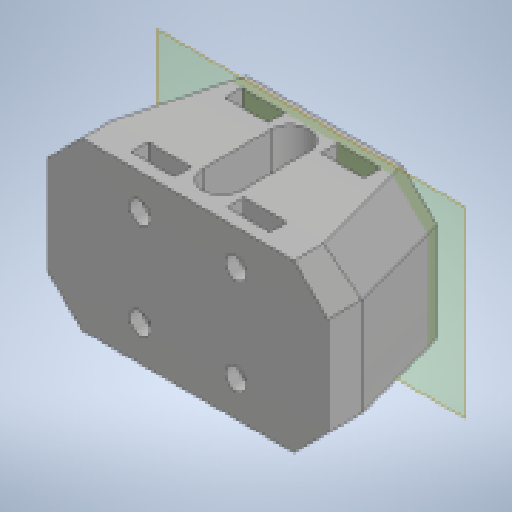
# Autodesk Inventor part: MCP-V
Saved by Autodesk Inventor 2026 (Build 300175050, 175E)
## iProperties
Created: 2025-12-08
Part Number: MCP-V
Material: Genérico
Document SubType Name: Modeling
Designer: user
Density: 1 g/cm^3
Appearance: Gris claro
Author: user
Autodesk Inventor part; units mm, degrees
ref_plane "YZ Plane" through (0, 0, 0) normal (1, 0, 0) x (0, 1, 0)
ref_plane "Plano de trabajo1" through (-13.3, -9.8, -7.75) normal (0, 0, 1) x (1, 0, 0)
ref_plane "Plano de trabajo2" through (-13.3, -9.8, -8.0345) normal (0, 0, 1) x (1, 0, 0)
sketch "Boceto1" plane through (0, 0, 0) normal (0, 0, 1) x (1, 0, 0)
  line L0 (13.3, 9.8) -> (-13.3, 9.8) projected
  line L1 (-13.3, -9.8) -> (-13.3, 9.8) projected
  line L2 (-13.3, -9.8) -> (13.3, -9.8) projected
  line L3 (13.3, 9.8) -> (13.3, -9.8) projected
  circle A0 centre (8, 8) radius 0.8 projected
  circle A1 centre (-8, -8) radius 0.8 projected
  circle A2 centre (-8, 8) radius 0.8 projected
  circle A3 centre (0, 0) radius 4 projected
  circle A4 centre (6, 0) radius 1.025 projected
  circle A5 centre (0, 6) radius 1.025 projected
  circle A6 centre (-6, 0) radius 1.025 projected
  circle A7 centre (0, -6) radius 1.025 projected
  circle A8 centre (5.6569, 5.6569) radius 1.025 projected
  circle A9 centre (-5.6569, 5.6569) radius 1.025 projected
  circle A10 centre (-5.6569, -5.6569) radius 1.025 projected
  circle A11 centre (5.6569, -5.6569) radius 1.025 projected
  circle A12 centre (9, -3) radius 1.025 projected
  circle A13 centre (9, 3) radius 1.025 projected
  circle A14 centre (-9, -3) radius 1.025 projected
  circle A15 centre (-9, 3) radius 1.025 projected
  circle A16 centre (8, -8) radius 0.8 projected
  circle A17 centre (-5.6569, -5.6569) radius 1.25
  circle A18 centre (5.6569, -5.6569) radius 1.25
  circle A19 centre (5.6569, 5.6569) radius 1.25
  circle A20 centre (-5.6569, 5.6569) radius 1.25
  line L4 (-16.5, -9.7) -> (-16.5, 9.7) projected
  line L5 (16.5, -9.7) -> (16.5, 9.7) projected
  line L6 (-13.3, -9.8) -> (-16.5, -9.8)
  line L7 (-13.3, 9.8) -> (-16.5, 9.8)
  line L8 (13.3, 9.8) -> (16.5, 9.8)
  line L9 (13.3, -9.8) -> (16.5, -9.8)
  line L10 (-16.5, -9.8) -> (-16.5, -9.7)
  line L11 (-16.5, 9.7) -> (-16.5, 9.8)
  line L12 (16.5, 9.8) -> (16.5, 9.7)
  line L13 (16.5, -9.8) -> (16.5, -9.7)
  point P0 (0, 0)
  dimension "d30" = 2.5
  constraints: 16 end point, 4 centre point, 4 collinear, 4 point on line, 3 equal length, 3 equal radius, 1 vertical
  measures "d30" diameter of A17
extrude "Extrusión1" add sketch "Boceto1" against normal up to surface (8.0345 mm away) contours L3 L2 L1 L0 | L8 L12 L5 L13 L9 L3 | L1 L6 L10 L4 L11 L7 | A0 | A1 | A2 | A3 | A4 | A5 | A6 | A7 | A12 | A13 | A14 | A15 | A16
ref_plane "Plano de trabajo3" through (16.5, 9.8, -6.5345) normal (0, 0, -1) x (-1, 0, 0)
sketch "Boceto2" plane through (0, 0, -6.5345) normal (0, 0, -1) x (-1, 0, 0)
  arc A0 (3.8297, -1.1547) -> (3.8297, 1.1547) centre (0, 0) ccw construction
  line L0 (3.8297, -1.1547) -> (4, -1.1547) construction
  line L1 (4, -1.1547) -> (4.7835, -1.6071) construction
  line L2 (4.7835, -1.6071) -> (4.8435, -1.5031) construction
  line L3 (4.8435, -1.5031) -> (5.2765, -1.7531) construction
  line L4 (5.2765, -1.7531) -> (5.2165, -1.8571) construction
  line L5 (5.2165, -1.8571) -> (6, -2.3094) construction
  line L6 (6, -2.3094) -> (6.55, -1.9919) construction
  arc A1 (7, -2.2517) -> (6.55, -1.9919) centre (6.7, -2.2517) ccw construction
  line L7 (7, -2.2517) -> (7, -2.75) construction
  line L8 (7, -2.75) -> (7.12, -2.75) construction
  line L9 (7.12, -2.75) -> (7.12, -3.25) construction
  line L10 (7.12, -3.25) -> (7, -3.25) construction
  line L11 (7, -3.25) -> (7, -4.1547) construction
  line L12 (7, -4.1547) -> (6.789, -4.3224) construction
  arc A2 (6.789, -4.3224) -> (7.2125, -4.8553) centre (5.6569, -5.6569) ccw construction
  line L13 (7.2125, -4.8553) -> (7.6337, -4.5206) construction
  line L14 (7.6337, -4.5206) -> (9, -5.3094) construction
  line L15 (9, -5.3094) -> (9.7835, -4.8571) construction
  line L16 (9.7835, -4.8571) -> (9.7235, -4.7531) construction
  line L17 (9.7235, -4.7531) -> (10.1565, -4.5031) construction
  line L18 (10.1565, -4.5031) -> (10.2165, -4.6071) construction
  line L19 (10.2165, -4.6071) -> (11, -4.1547) construction
  line L20 (11, -4.1547) -> (11, -1.8453) construction
  line L21 (11, -1.8453) -> (10.2165, -1.3929) construction
  line L22 (10.2165, -1.3929) -> (10.1565, -1.4969) construction
  line L23 (10.1565, -1.4969) -> (9.7235, -1.2469) construction
  line L24 (9.7235, -1.2469) -> (9.7835, -1.1429) construction
  line L25 (9.7835, -1.1429) -> (9, -0.6906) construction
  line L26 (9, -0.6906) -> (8.45, -1.0081) construction
  arc A3 (8, -0.7483) -> (8.45, -1.0081) centre (8.3, -0.7483) ccw construction
  line L27 (8, -0.7483) -> (8, -0.25) construction
  line L28 (8, -0.25) -> (7.88, -0.25) construction
  line L29 (7.88, -0.25) -> (7.88, 0.25) construction
  line L30 (7.88, 0.25) -> (8, 0.25) construction
  line L31 (8, 0.25) -> (8, 0.7483) construction
  arc A4 (8.45, 1.0081) -> (8, 0.7483) centre (8.3, 0.7483) ccw construction
  line L32 (8.45, 1.0081) -> (9, 0.6906) construction
  line L33 (9, 0.6906) -> (9.7835, 1.1429) construction
  line L34 (9.7835, 1.1429) -> (9.7235, 1.2469) construction
  line L35 (9.7235, 1.2469) -> (10.1565, 1.4969) construction
  line L36 (10.1565, 1.4969) -> (10.2165, 1.3929) construction
  line L37 (10.2165, 1.3929) -> (11, 1.8453) construction
  line L38 (11, 1.8453) -> (11, 4.1547) construction
  line L39 (11, 4.1547) -> (10.2165, 4.6071) construction
  line L40 (10.2165, 4.6071) -> (10.1565, 4.5031) construction
  line L41 (10.1565, 4.5031) -> (9.7235, 4.7531) construction
  line L42 (9.7235, 4.7531) -> (9.7835, 4.8571) construction
  line L43 (9.7835, 4.8571) -> (9, 5.3094) construction
  line L44 (9, 5.3094) -> (7.6337, 4.5206) construction
  line L45 (7.6337, 4.5206) -> (7.2125, 4.8553) construction
  arc A5 (7.2125, 4.8553) -> (6.789, 4.3224) centre (5.6569, 5.6569) ccw construction
  line L46 (6.789, 4.3224) -> (7, 4.1547) construction
  line L47 (7, 4.1547) -> (7, 3.25) construction
  line L48 (7, 3.25) -> (7.12, 3.25) construction
  line L49 (7.12, 3.25) -> (7.12, 2.75) construction
  line L50 (7.12, 2.75) -> (7, 2.75) construction
  line L51 (7, 2.75) -> (7, 2.2517) construction
  arc A6 (6.55, 1.9919) -> (7, 2.2517) centre (6.7, 2.2517) ccw construction
  line L52 (6.55, 1.9919) -> (6, 2.3094) construction
  line L53 (6, 2.3094) -> (5.2165, 1.8571) construction
  line L54 (5.2165, 1.8571) -> (5.2765, 1.7531) construction
  line L55 (5.2765, 1.7531) -> (4.8435, 1.5031) construction
  line L56 (4.8435, 1.5031) -> (4.7835, 1.6071) construction
  line L57 (4.7835, 1.6071) -> (4, 1.1547) construction
  line L58 (4, 1.1547) -> (3.8297, 1.1547) construction
  circle A7 centre (6, 0) radius 1.025 construction
  circle A8 centre (5.6569, 5.6569) radius 1.025 construction
  circle A9 centre (5.6569, -5.6569) radius 1.025 construction
  circle A10 centre (9, -3) radius 1.025 construction
  circle A11 centre (9, 3) radius 1.025 construction
  line L59 (-4.5022, 7.6569) -> (-3.3475, 5.6569) construction
  line L60 (-3.3475, 5.6569) -> (-4.5022, 3.6569) construction
  line L61 (-4.5022, 3.6569) -> (-6.8116, 3.6569) construction
  line L62 (-6.8116, 3.6569) -> (-7.9663, 5.6569) construction
  line L63 (-7.9663, 5.6569) -> (-6.8116, 7.6569) construction
  line L64 (-6.8116, 7.6569) -> (-4.5022, 7.6569) construction
  arc A12 (-3.8297, -1.1547) -> (-3.8297, 1.1547) centre (0, 0) ccw construction
  line L65 (-3.8297, 1.1547) -> (-4, 1.1547) construction
  line L66 (-4, 1.1547) -> (-4.7835, 1.6071) construction
  line L67 (-4.7835, 1.6071) -> (-4.8435, 1.5031) construction
  line L68 (-4.8435, 1.5031) -> (-5.2765, 1.7531) construction
  line L69 (-5.2765, 1.7531) -> (-5.2165, 1.8571) construction
  line L70 (-5.2165, 1.8571) -> (-6, 2.3094) construction
  line L71 (-6, 2.3094) -> (-6.55, 1.9919) construction
  arc A13 (-7, 2.2517) -> (-6.55, 1.9919) centre (-6.7, 2.2517) ccw construction
  line L72 (-7, 2.2517) -> (-7, 2.75) construction
  line L73 (-7, 2.75) -> (-7.12, 2.75) construction
  line L74 (-7.12, 2.75) -> (-7.12, 3.25) construction
  line L75 (-7.12, 3.25) -> (-7, 3.25) construction
  line L76 (-7, 3.25) -> (-7, 4.1547) construction
  line L77 (-7, 4.1547) -> (-6.789, 4.3224) construction
  arc A14 (-6.789, 4.3224) -> (-7.2125, 4.8553) centre (-5.6569, 5.6569) ccw construction
  line L78 (-7.2125, 4.8553) -> (-7.6337, 4.5206) construction
  line L79 (-7.6337, 4.5206) -> (-9, 5.3094) construction
  line L80 (-9, 5.3094) -> (-9.7835, 4.8571) construction
  line L81 (-9.7835, 4.8571) -> (-9.7235, 4.7531) construction
  line L82 (-9.7235, 4.7531) -> (-10.1565, 4.5031) construction
  line L83 (-10.1565, 4.5031) -> (-10.2165, 4.6071) construction
  line L84 (-10.2165, 4.6071) -> (-11, 4.1547) construction
  line L85 (-11, 4.1547) -> (-11, 1.8453) construction
  line L86 (-11, 1.8453) -> (-10.2165, 1.3929) construction
  line L87 (-10.2165, 1.3929) -> (-10.1565, 1.4969) construction
  line L88 (-10.1565, 1.4969) -> (-9.7235, 1.2469) construction
  line L89 (-9.7235, 1.2469) -> (-9.7835, 1.1429) construction
  line L90 (-9.7835, 1.1429) -> (-9, 0.6906) construction
  line L91 (-9, 0.6906) -> (-8.45, 1.0081) construction
  arc A15 (-8, 0.7483) -> (-8.45, 1.0081) centre (-8.3, 0.7483) ccw construction
  line L92 (-8, 0.7483) -> (-8, 0.25) construction
  line L93 (-8, 0.25) -> (-7.88, 0.25) construction
  line L94 (-7.88, 0.25) -> (-7.88, -0.25) construction
  line L95 (-7.88, -0.25) -> (-8, -0.25) construction
  line L96 (-8, -0.25) -> (-8, -0.7483) construction
  arc A16 (-8.45, -1.0081) -> (-8, -0.7483) centre (-8.3, -0.7483) ccw construction
  line L97 (-8.45, -1.0081) -> (-9, -0.6906) construction
  line L98 (-9, -0.6906) -> (-9.7835, -1.1429) construction
  line L99 (-9.7835, -1.1429) -> (-9.7235, -1.2469) construction
  line L100 (-9.7235, -1.2469) -> (-10.1565, -1.4969) construction
  line L101 (-10.1565, -1.4969) -> (-10.2165, -1.3929) construction
  line L102 (-10.2165, -1.3929) -> (-11, -1.8453) construction
  line L103 (-11, -1.8453) -> (-11, -4.1547) construction
  line L104 (-11, -4.1547) -> (-10.2165, -4.6071) construction
  line L105 (-10.2165, -4.6071) -> (-10.1565, -4.5031) construction
  line L106 (-10.1565, -4.5031) -> (-9.7235, -4.7531) construction
  line L107 (-9.7235, -4.7531) -> (-9.7835, -4.8571) construction
  line L108 (-9.7835, -4.8571) -> (-9, -5.3094) construction
  line L109 (-9, -5.3094) -> (-7.6337, -4.5206) construction
  line L110 (-7.6337, -4.5206) -> (-7.2125, -4.8553) construction
  arc A17 (-7.2125, -4.8553) -> (-6.789, -4.3224) centre (-5.6569, -5.6569) ccw construction
  line L111 (-6.789, -4.3224) -> (-7, -4.1547) construction
  line L112 (-7, -4.1547) -> (-7, -3.25) construction
  line L113 (-7, -3.25) -> (-7.12, -3.25) construction
  line L114 (-7.12, -3.25) -> (-7.12, -2.75) construction
  line L115 (-7.12, -2.75) -> (-7, -2.75) construction
  line L116 (-7, -2.75) -> (-7, -2.2517) construction
  arc A18 (-6.55, -1.9919) -> (-7, -2.2517) centre (-6.7, -2.2517) ccw construction
  line L117 (-6.55, -1.9919) -> (-6, -2.3094) construction
  line L118 (-6, -2.3094) -> (-5.2165, -1.8571) construction
  line L119 (-5.2165, -1.8571) -> (-5.2765, -1.7531) construction
  line L120 (-5.2765, -1.7531) -> (-4.8435, -1.5031) construction
  line L121 (-4.8435, -1.5031) -> (-4.7835, -1.6071) construction
  line L122 (-4.7835, -1.6071) -> (-4, -1.1547) construction
  line L123 (-4, -1.1547) -> (-3.8297, -1.1547) construction
  circle A19 centre (-6, 0) radius 1.025 construction
  circle A20 centre (-5.6569, 5.6569) radius 1.025 construction
  circle A21 centre (-5.6569, -5.6569) radius 1.025 construction
  circle A22 centre (-9, -3) radius 1.025 construction
  circle A23 centre (-9, 3) radius 1.025 construction
  line L124 (-6.927, 7.8569) -> (-8.1972, 5.6569)
  line L125 (-8.1972, 5.6569) -> (-6.927, 3.4569)
  line L126 (-6.927, 3.4569) -> (-4.3867, 3.4569)
  line L127 (-4.3867, 3.4569) -> (-3.1165, 5.6569)
  line L128 (-3.1165, 5.6569) -> (-4.3867, 7.8569)
  line L129 (-4.3867, 7.8569) -> (-6.927, 7.8569)
  line L130 (-16.5, 9.8) -> (16.5, 9.8) projected
  line L131 (16.5, 9.8) -> (16.5, -9.8) projected
  line L132 (16.5, -9.8) -> (-16.5, -9.8) projected
  line L133 (-16.5, -9.8) -> (-16.5, 9.8) projected
  circle A24 centre (5.6569, -5.6569) radius 1.25 projected
  circle A25 centre (-5.6569, -5.6569) radius 1.25 projected
  circle A26 centre (-5.6569, 5.6569) radius 1.25 projected
  circle A27 centre (5.6569, 5.6569) radius 1.25 projected
  line L134 (-8.1972, 5.6569) -> (-8.1972, 9.8)
  line L135 (-3.1165, 5.6569) -> (-3.1165, 9.8)
  line L136 (0, 9.8) -> (0, -9.8) construction
  line L137 (-16.5, 0) -> (16.5, 0) construction
  line L138 (16.5, 9.8) -> (16.5, -9.8) projected
  line L139 (6.927, 7.8569) -> (8.1972, 5.6569)
  line L140 (8.1972, 5.6569) -> (6.927, 3.4569)
  line L141 (6.927, 3.4569) -> (4.3867, 3.4569)
  line L142 (4.3867, 3.4569) -> (3.1165, 5.6569)
  line L143 (3.1165, 5.6569) -> (4.3867, 7.8569)
  line L144 (4.3867, 7.8569) -> (6.927, 7.8569)
  line L145 (8.1972, 5.6569) -> (8.1972, 9.8)
  line L146 (3.1165, 5.6569) -> (3.1165, 9.8)
  line L147 (-6.927, -7.8569) -> (-8.1972, -5.6569)
  line L148 (-8.1972, -5.6569) -> (-6.927, -3.4569)
  line L149 (-6.927, -3.4569) -> (-4.3867, -3.4569)
  line L150 (-4.3867, -3.4569) -> (-3.1165, -5.6569)
  line L151 (-3.1165, -5.6569) -> (-4.3867, -7.8569)
  line L152 (-4.3867, -7.8569) -> (-6.927, -7.8569)
  line L153 (-8.1972, -5.6569) -> (-8.1972, -9.8)
  line L154 (-3.1165, -5.6569) -> (-3.1165, -9.8)
  line L155 (8.1972, -5.6569) -> (8.1972, -9.8)
  line L156 (6.927, -7.8569) -> (8.1972, -5.6569)
  line L157 (8.1972, -5.6569) -> (6.927, -3.4569)
  line L158 (6.927, -3.4569) -> (4.3867, -3.4569)
  line L159 (4.3867, -3.4569) -> (3.1165, -5.6569)
  line L160 (3.1165, -5.6569) -> (3.1165, -9.8)
  line L161 (3.1165, -5.6569) -> (4.3867, -7.8569)
  line L162 (4.3867, -7.8569) -> (6.927, -7.8569)
  point P0 (-8.1972, -9.8)
  point P1 (-3.1165, -9.8)
  point P2 (3.1165, -9.8)
  point P3 (8.1972, -9.8)
  point P4 (0, 0)
  dimension "d3" = 4.6188
  dimension "d103" = 0.2
  constraints: 80 end point, 24 symmetric about line, 6 midpoint, 3 perpendicular, 2 point on line, 1 coincident, 1 horizontal, 1 parallel, 18 other
  measures "d3" distance of L59.end L62.end
  measures "d103" distance between parallel lines of L63 L124
extrude "Extrusión2" cut sketch "Boceto2" against normal blind 2 contours L129 L128 L127 L126 L125 L124 | L124 L134 L130 L135 L128 L129 | L130 L145 L139 L144 L143 L146 | L153 L147 L152 L151 L154 L132 | L143 L144 L139 L140 L141 L142 | L148 L149 L150 L151 L152 L147 | L160 L161 L162 L156 L155 L132 | L159 L158 L157 L156 L162 L161 | A24 | A25 | A26 | A27
mirror "Simetría3" about plane through (0, 0, 0) normal (0, 0, 1)
chamfer "Chaflán2" distance 3.2 distance2 12.069 2 edges at (16.5, 0, -8.0345) (-16.5, 0, -8.0345) measured on face at (16, 0, -8.0345) measured on face at (-16, 0, -8.0345)
chamfer "Chaflán6" distance 4 angle 45 8 edges at (14.9, 9.8, -2) (16.5, 9.8, 6.0345) (14.9, -9.8, -2) (16.5, -9.8, 6.0345) (-14.9, -9.8, -2) (-16.5, -9.8, 6.0345) (-14.9, 9.8, -2) (-16.5, 9.8, 6.0345)
sketch "Boceto6" plane through (0, 0, 0) normal (0, 1, 0) x (-1, 0, 0)
  line L0 (0, 4) -> (0, -4) construction
  line L1 (-2.25, 4) -> (-2.25, -4)
  line L2 (2.25, -4) -> (2.25, 4)
  arc A0 (2.25, 4) -> (-2.25, 4) centre (0, 4) ccw
  arc A1 (-2.25, -4) -> (2.25, -4) centre (0, -4) ccw
  point P0 (0, 0)
  point P1 (0, 6.25)
  point P2 (0, -6.25)
  dimension "d95" = 4.5
  dimension "d96" = 12.5
  constraints: 8 end point, 6 point on circle, 4 tangent, 2 centre point, 1 midpoint, 1 parallel, 1 vertical
  measures "d95" diameter of A1
  measures "d96" distance of point (0, 6.25) point (0, -6.25)
extrude "Extrusión5" cut sketch "Boceto6" along normal through all both and the other way through all
equation "\"d3\" = d2"
equation "\"d2\" = 4.618802"
